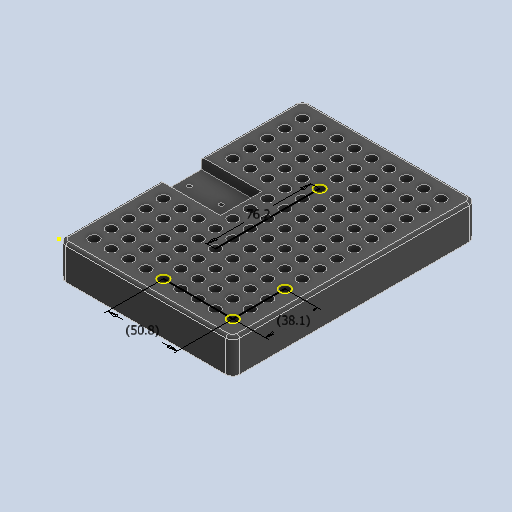
# Autodesk Inventor part: Base
Saved by Autodesk Inventor 2026 (Build 300175050, 175E)
## iProperties
Created: 2025-09-26
Part Number: Base
Material: Plastico PETG
Document SubType Name: Modeling
Designer: bello
Density: 1.27 g/cm^3
Appearance: Genérico
Author: bello
Autodesk Inventor part; units mm, degrees
ref_plane "YZ Plane" through (0, 0, 0) normal (1, 0, 0) x (0, 1, 0)
ref_plane "XZ Plane" through (0, 0, 0) normal (0, 1, 0) x (-1, 0, 0)
ref_plane "XY Plane" through (0, 0, 0) normal (0, 0, 1) x (1, 0, 0)
sketch "Boceto1" plane through (0, 0, 0) normal (0, 1, 0) x (-1, 0, 0)
  line L0 (0, 0) -> (-127, 0)
  line L1 (-127, 0) -> (-127, -178)
  line L2 (-127, -178) -> (0, -178)
  line L3 (0, -178) -> (0, 0)
  dimension "d0" = 127
  dimension "d1" = 178
  constraints: 8 end point, 2 parallel, 1 horizontal, 1 perpendicular
  measures "d0" distance of L1.end L2.end
  measures "d1" distance of L2.end L0.start
extrude "Extrusión1" add sketch "Boceto1" along normal blind 25
fillet "Empalme1" radius 5 4 edges at (127, 12.5, 0) (0, 12.5, 0) (127, 12.5, -178) (0, 12.5, -178)
sketch "Boceto2" plane through (0, 25, 0) normal (0, 1, 0) x (1, 0, 0)
  circle A0 centre (114.3, 12.8) radius 3.7
  line L0 (5, 0) -> (122, 0) projected
  line L1 (127, 5) -> (127, 173) projected
  line L2 (114.3, 12.8) -> (114.3, 212.2204)
  line L3 (114.3, 12.8) -> (-11.6799, 12.8)
  line L4 (122, 178) -> (5, 178) projected
  line L5 (-9.217, 89) -> (159.5001, 89)
  circle A1 centre (114.3, 25.5) radius 3.7
  circle A2 centre (114.3, 38.2) radius 3.7
  circle A3 centre (114.3, 50.9) radius 3.7
  circle A4 centre (114.3, 63.6) radius 3.7
  circle A5 centre (114.3, 76.3) radius 3.7
  circle A6 centre (114.3, 89) radius 3.7
  circle A7 centre (114.3, 101.7) radius 3.7
  circle A8 centre (114.3, 114.4) radius 3.7
  circle A9 centre (114.3, 127.1) radius 3.7
  circle A10 centre (114.3, 139.8) radius 3.7
  circle A11 centre (114.3, 152.5) radius 3.7
  circle A12 centre (114.3, 165.2) radius 3.7
  line L6 (63.5, -14.924) -> (63.5, 199.6475)
  circle A13 centre (101.6, 12.8) radius 3.7
  circle A14 centre (101.6, 89) radius 3.7
  circle A15 centre (101.6, 101.7) radius 3.7
  circle A16 centre (101.6, 114.4) radius 3.7
  circle A17 centre (101.6, 127.1) radius 3.7
  circle A18 centre (101.6, 139.8) radius 3.7
  circle A19 centre (101.6, 152.5) radius 3.7
  circle A20 centre (101.6, 165.2) radius 3.7
  circle A21 centre (101.6, 63.6) radius 3.7
  circle A22 centre (101.6, 50.9) radius 3.7
  circle A23 centre (101.6, 38.2) radius 3.7
  circle A24 centre (101.6, 25.5) radius 3.7
  circle A25 centre (101.6, 76.3) radius 3.7
  circle A26 centre (88.9, 12.8) radius 3.7
  circle A27 centre (88.9, 89) radius 3.7
  circle A28 centre (88.9, 101.7) radius 3.7
  circle A29 centre (88.9, 114.4) radius 3.7
  circle A30 centre (88.9, 127.1) radius 3.7
  circle A31 centre (88.9, 139.8) radius 3.7
  circle A32 centre (88.9, 152.5) radius 3.7
  circle A33 centre (88.9, 165.2) radius 3.7
  circle A34 centre (88.9, 63.6) radius 3.7
  circle A35 centre (88.9, 50.9) radius 3.7
  circle A36 centre (88.9, 38.2) radius 3.7
  circle A37 centre (88.9, 25.5) radius 3.7
  circle A38 centre (88.9, 76.3) radius 3.7
  circle A39 centre (76.2, 12.8) radius 3.7
  circle A40 centre (76.2, 89) radius 3.7
  circle A41 centre (76.2, 101.7) radius 3.7
  circle A42 centre (76.2, 114.4) radius 3.7
  circle A43 centre (76.2, 127.1) radius 3.7
  circle A44 centre (76.2, 139.8) radius 3.7
  circle A45 centre (76.2, 152.5) radius 3.7
  circle A46 centre (76.2, 165.2) radius 3.7
  circle A47 centre (76.2, 63.6) radius 3.7
  circle A48 centre (76.2, 50.9) radius 3.7
  circle A49 centre (76.2, 38.2) radius 3.7
  circle A50 centre (76.2, 25.5) radius 3.7
  circle A51 centre (76.2, 76.3) radius 3.7
  circle A52 centre (63.5, 12.8) radius 3.7
  circle A53 centre (63.5, 89) radius 3.7
  circle A54 centre (63.5, 101.7) radius 3.7
  circle A55 centre (63.5, 114.4) radius 3.7
  circle A56 centre (63.5, 127.1) radius 3.7
  circle A57 centre (63.5, 139.8) radius 3.7
  circle A58 centre (63.5, 152.5) radius 3.7
  circle A59 centre (63.5, 165.2) radius 3.7
  circle A60 centre (63.5, 63.6) radius 3.7
  circle A61 centre (63.5, 50.9) radius 3.7
  circle A62 centre (63.5, 38.2) radius 3.7
  circle A63 centre (63.5, 25.5) radius 3.7
  circle A64 centre (63.5, 76.3) radius 3.7
  circle A65 centre (50.8, 12.8) radius 3.7
  circle A66 centre (50.8, 89) radius 3.7
  circle A67 centre (50.8, 101.7) radius 3.7
  circle A68 centre (50.8, 114.4) radius 3.7
  circle A69 centre (50.8, 127.1) radius 3.7
  circle A70 centre (50.8, 139.8) radius 3.7
  circle A71 centre (50.8, 152.5) radius 3.7
  circle A72 centre (50.8, 165.2) radius 3.7
  circle A73 centre (50.8, 63.6) radius 3.7
  circle A74 centre (50.8, 50.9) radius 3.7
  circle A75 centre (50.8, 38.2) radius 3.7
  circle A76 centre (50.8, 25.5) radius 3.7
  circle A77 centre (50.8, 76.3) radius 3.7
  circle A78 centre (38.1, 63.6) radius 3.7
  circle A79 centre (38.1, 50.9) radius 3.7
  circle A80 centre (38.1, 38.2) radius 3.7
  circle A81 centre (38.1, 25.5) radius 3.7
  circle A82 centre (38.1, 12.8) radius 3.7
  circle A83 centre (38.1, 165.2) radius 3.7
  circle A84 centre (38.1, 152.5) radius 3.7
  circle A85 centre (38.1, 139.8) radius 3.7
  circle A86 centre (38.1, 127.1) radius 3.7
  circle A87 centre (38.1, 114.4) radius 3.7
  circle A88 centre (25.4, 63.6) radius 3.7
  circle A89 centre (25.4, 50.9) radius 3.7
  circle A90 centre (25.4, 38.2) radius 3.7
  circle A91 centre (25.4, 25.5) radius 3.7
  circle A92 centre (25.4, 12.8) radius 3.7
  circle A93 centre (25.4, 165.2) radius 3.7
  circle A94 centre (25.4, 152.5) radius 3.7
  circle A95 centre (25.4, 139.8) radius 3.7
  circle A96 centre (25.4, 127.1) radius 3.7
  circle A97 centre (25.4, 114.4) radius 3.7
  circle A98 centre (12.7, 63.6) radius 3.7
  circle A99 centre (12.7, 50.9) radius 3.7
  circle A100 centre (12.7, 38.2) radius 3.7
  circle A101 centre (12.7, 25.5) radius 3.7
  circle A102 centre (12.7, 12.8) radius 3.7
  circle A103 centre (12.7, 165.2) radius 3.7
  circle A104 centre (12.7, 152.5) radius 3.7
  circle A105 centre (12.7, 139.8) radius 3.7
  circle A106 centre (12.7, 127.1) radius 3.7
  circle A107 centre (12.7, 114.4) radius 3.7
  point P0 (0, 0)
  point P1 (107.6319, 178)
  point P2 (114.3, 92.7)
  point P3 (114.3, 85.3)
  point P4 (114.3, 105.4)
  point P5 (114.3, 98)
  dimension "d5" = 7.4
  dimension "d100" = 12.7
  dimension "d105" = 152.4
  dimension "d106" = 152.4
  dimension "d110" = 12.7
  dimension "d117" = 12.7
  dimension "d122" = 101.6
  dimension "d123" = 101.6
  constraints: 108 centre point, 8 end point, 5 horizontal, 3 vertical, 214 other
  measures "d5" diameter of A0
  measures "d100" distance of L2.start A1.centre
  measures "d105" distance of A12.centre L2.start
  measures "d106" diameter of L2.start L5
  measures "d110" distance of L2.start A13.centre
  measures "d117" distance of A73.centre A78.centre
  measures "d122" distance of L2.start A102.centre
  measures "d123" diameter of L2.start L6
extrude "Extrusión2" cut sketch "Boceto2" against normal blind 12.7 contours A0 L3 L2 | A102 L3 | L3 A102 | A92 L3 | L3 A92 | A82 L3 | L3 A82 | A65 L3 | L3 A65 | A66 L5 | L5 A66 | L2 L3 A0 | A1 L2 | L2 A1 | A13 L3 | L3 A13 | A2 L2 | L2 A2 | A26 L3 | L3 A26 | A3 L2 | L2 A3 | A39 L3 | L3 A39 | A4 L2 | L2 A4 | A52 L6 L3 | L3 L6 A52 | L6 A52 L3 | L3 A52 L6 | A5 L2 | L2 A5 | A63 L6 | L6 A63 | A6 L5 L2 | L2 L5 A6 | A62 L6 | L6 A62 | L5 A6 L2 | L2 A6 L5 | A14 L5 | L5 A14 | A61 L6 | L6 A61 | A7 L2 | L2 A7 | A27 L5 | L5 A27 | A60 L6 | L6 A60 | A8 L2 | L2 A8 | A40 L5 | L5 A40 | A64 L6 | L6 A64 | A9 L2 | L2 A9 | A53 L6 L5 | L5 L6 A53 | A53 L5 L6 | A10 L2 | L2 A10 | L5 A53 L6 | A54 L6 | L6 A54 | A11 L2 | L2 A11 | A55 L6 | L6 A55 | A12 L2 | L2 A12 | A56 L6 | L6 A56 | A57 L6 | L6 A57 | A59 L6 | L6 A59 | A58 L6 | L6 A58 | A15 | A16 | A17 | A18 | A19 | A20 | A21 | A22 | A23 | A24 | A25 | A28 | A29 | A30 | A31 | A32 | A33 | A34 | A35 | A36 | A37 | A38 | A41 | A42 | A43 | A44 | A45 | A46 | A47 | A48 | A49 | A50 | A51 | A67 | A68 | A69 | A70 | A71 | A72 | A73 | A74 | A75 | A76 | A77 | A78 | A79 | A80 | A81 | A83 | A84 | A85 | A86 | A87 | A88 | A89 | A90 | A91 | A93 | A94 | A95 | A96 | A97 | A98 | A99 | A100 | A101 | A103 | A104 | A105 | A106 | A107
sketch "Boceto3" plane through (0, 25, 0) normal (0, 1, 0) x (1, 0, 0)
  line L0 (-9.0869, 89) -> (43.2894, 89)
  line L1 (44.2, 73.85) -> (44.2, 89)
  line L2 (44.2, 104.15) -> (0, 104.15)
  line L3 (44.2, 104.15) -> (44.2, 89)
  line L4 (0, 104.15) -> (0, 89)
  line L5 (0, 89) -> (0, 73.85)
  line L6 (0, 73.85) -> (44.2, 73.85)
  point P0 (0, 0)
  point P1 (0, 89)
  dimension "d39" = 44.2
  dimension "d40" = 15.15
  dimension "d41" = 15.15
  constraints: 14 end point, 5 perpendicular, 4 point on line, 2 horizontal, 1 other
  measures "d39" distance of L2.start L2.end
  measures "d40" distance of L2.end L4.end
  measures "d41" distance of L4.end L5.end
extrude "Extrusión3" cut sketch "Boceto3" against normal blind 8
sketch "Boceto4" plane through (0, 0, 0) normal (0, -1, 0) x (1, 0, 0)
  line L0 (-20.4623, -89) -> (73.7948, -89)
  circle A0 centre (6.2, -89) radius 3.25
  circle A1 centre (29.5, -89) radius 3.25
  line L1 (0, -173) -> (0, -5) projected
  point P0 (0, 0)
  dimension "d44" = 6.5
  dimension "d45" = 6.5
  dimension "d46" = 6.2
  dimension "d47" = 23.3
  constraints: 2 centre point, 2 end point, 2 horizontal, 2 point on line
  measures "d44" diameter of A1
  measures "d45" diameter of A0
  measures "d46" distance from line of L1 A0.centre
  measures "d47" distance of A1.centre A0.centre
extrude "Extrusión4" cut sketch "Boceto4" against normal blind 12
sketch "Boceto5" plane through (29.5, 12, -89) normal (0, -1, 0) x (1, 0, 0)
  circle A0 centre (-23.3, 0) radius 3.25 projected
  circle A1 centre (-23.3, 0) radius 1.6
  circle A2 centre (0, 0) radius 3.25 projected
  circle A3 centre (0, 0) radius 1.6
  point P0 (-29.5, 89)
  dimension "d50" = 3.2
  dimension "d51" = 3.2
  constraints: 2 centre point, 2 coincident
  measures "d50" diameter of A3
  measures "d51" diameter of A1
extrude "Extrusión5" cut sketch "Boceto5" against normal blind 14.5 contours A1 | A3
fillet "Empalme2" radius 2 9 edges at (1.4645, 25, -176.5355) (63.5, 25, -178) (125.5355, 25, -176.5355) (127, 25, -89) (125.5355, 25, -1.4645) (63.5, 25, 0) (1.4645, 25, -1.4645) (0, 25, -39.425) (0, 25, -138.575)
sketch "Boceto6" plane through (0, 0, 0) normal (0, -1, 0) x (1, 0, 0)
  line L0 (139.3096, -89) -> (-15.7113, -89)
  line L1 (127, -5) -> (127, -173) projected
  line L2 (127, -89) -> (106, -89)
  line L3 (106, -89) -> (106, -81)
  line L4 (127, -81.5) -> (127, -89)
  line L5 (127, -89) -> (106, -89)
  line L6 (106, -89) -> (106, -97)
  line L7 (106, -97) -> (127, -97)
  line L8 (127, -97) -> (127, -89)
  line L9 (106, -81) -> (124, -81)
  line L10 (124, -81) -> (124, -97)
  line L11 (124, -97) -> (106, -97)
  line L12 (106, -97) -> (106, -81)
  point P0 (0, 0)
  dimension "d55" = 8
  dimension "d56" = 8
  dimension "d57" = 21
  dimension "d58" = 18
  constraints: 24 end point, 5 horizontal, 5 parallel, 3 perpendicular, 2 point on line, 1 midpoint
  measures "d55" distance of L2.end L3.end
  measures "d56" distance of L5.end L6.end
  measures "d57" distance of L6.end L7.end
  measures "d58" distance of L3.end L9.end
extrude "Extrusión6" cut sketch "Boceto6" against normal blind 13 contours L10 L7 L6 L0 | L0 L3 L9 L10
sketch "Boceto7" plane through (0, 25, 0) normal (0, 1, 0) x (1, 0, 0)
  circle A0 centre (114.3, 12.8) radius 3.7 projected
  circle A1 centre (114.3, 50.9) radius 3.7 projected
  line L0 (114.3, 12.8) -> (114.3, 50.9)
  circle A2 centre (63.5, 12.8) radius 3.7 projected
  line L1 (114.3, 12.8) -> (63.5, 12.8)
  circle A3 centre (63.5, 127.1) radius 3.7 projected
  line L2 (63.5, 50.9) -> (63.5, 127.1)
  point P0 (0, 0)
  dimension "d124" = 50.8
  dimension "d125" = 38.1
  dimension "d126" = 76.2
  constraints: 6 end point, 2 vertical, 1 horizontal
  measures "d124" distance of L0.start L1.end
  measures "d125" distance of L0.start L0.end
  measures "d126" distance of L2.start L2.end
equation "\"d30\" = d110"
